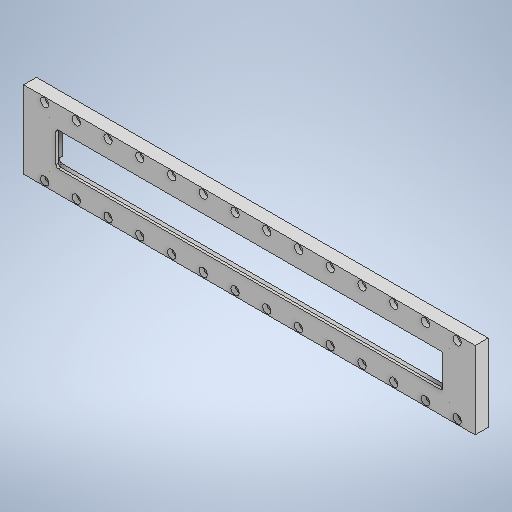
# Autodesk Inventor part: Bauteil4
Saved by Autodesk Inventor 2025.2 (Build 292293000, 293)
## iProperties
Created: 2025-01-07
Part Number: Bauteil4
Material: Generisch
Document SubType Name: Modeling
Designer: gorenfl4
Density: 1 g/cm^3
Appearance: Vorgabe
Author: gorenfl4
Autodesk Inventor part; units mm, degrees
ref_plane "YZ Plane" through (0, 0, 0) normal (1, 0, 0) x (0, 1, 0)
ref_plane "XZ Plane" through (0, 0, 0) normal (0, 1, 0) x (-1, 0, 0)
ref_plane "XY Plane" through (0, 0, 0) normal (0, 0, 1) x (1, 0, 0)
sketch "Skizze1" plane through (0, 0, 0) normal (0, 1, 0) x (-1, 0, 0)
  line L0 (0, 42.9058) -> (-350, 42.9058)
  line L1 (-350, 42.9058) -> (-350, -17.0942)
  line L2 (-350, -17.0942) -> (0, -17.0942)
  line L3 (0, -17.0942) -> (0, 42.9058)
  point P0 (0, 0)
  dimension "d0" = 350
  dimension "d1" = 0
  dimension "d2" = 60
  constraints: 8 end point, 2 parallel, 1 horizontal, 1 perpendicular
  measures "d0" distance from line of point (0, 0) L1
  measures "d1" distance from line of point (0, 0) L3
  measures "d2" distance between parallel lines of L0 L2
extrude "Extrusion1" add sketch "Skizze1" along normal blind 10
sketch "Skizze2" plane through (0, 10, 0) normal (0, 1, 0) x (1, 0, 0)
  line L0 (25, 0.0942) -> (325, 0.0942)
  line L1 (325, 0.0942) -> (325, -25.9058)
  line L2 (325, -25.9058) -> (25, -25.9058)
  line L3 (25, -25.9058) -> (25, 0.0942)
  line L4 (0, 17.0942) -> (0, -42.9058) projected
  line L5 (350, -42.9058) -> (350, 17.0942) projected
  line L6 (350, 17.0942) -> (0, 17.0942) projected
  line L7 (0, -42.9058) -> (350, -42.9058) projected
  point P0 (0, 0)
  point P1 (175, 17.0942)
  dimension "d5" = 25
  dimension "d6" = 25
  dimension "d7" = 17
  dimension "d8" = 17
  constraints: 8 end point, 2 parallel, 1 horizontal, 1 midpoint, 1 perpendicular
  measures "d5" distance between parallel lines of L4 L3
  measures "d6" distance between parallel lines of L5 L1
  measures "d7" distance from line of point (175, 17.094) L0
  measures "d8" distance between parallel lines of L7 L2
extrude "Extrusion2" cut sketch "Skizze2" against normal through all contours L0 L1 L2 L3
fillet "Rundung1" radius 2 1 edges at (25, 5, -0.0942)
fillet "Rundung2" radius 2 1 edges at (25, 5, 25.9058)
fillet "Rundung3" radius 2 1 edges at (325, 5, -0.0942)
fillet "Rundung4" radius 2 1 edges at (325, 5, 25.9058)
sketch "Skizze4" plane through (0, 10, 0) normal (0, 1, 0) x (1, 0, 0)
  line L0 (20, -30.9058) -> (330, -30.9058)
  line L1 (330, 5.0942) -> (20, 5.0942)
  line L2 (25, -23.9058) -> (25, -1.9058) projected
  line L3 (323, -25.9058) -> (27, -25.9058) projected
  line L4 (27, 0.0942) -> (323, 0.0942) projected
  line L5 (325, -1.9058) -> (325, -23.9058) projected
  arc A0 (20, 5.0942) -> (20, 0.0942) centre (20, 2.5942) ccw
  arc A1 (20, -25.9058) -> (20, -30.9058) centre (20, -28.4058) ccw
  arc A2 (330, 0.0942) -> (330, 5.0942) centre (330, 2.5942) ccw
  arc A3 (330, -30.9058) -> (330, -25.9058) centre (330, -28.4058) ccw
  line L6 (330, 0.0942) -> (330, -25.9058)
  line L7 (20, 0.0942) -> (20, -25.9058)
  point P0 (0, 0)
  dimension "d32" = 5
  dimension "d33" = 5
  dimension "d110" = 2.5
  dimension "d111" = 2.5
  dimension "d112" = 2.5
  dimension "d113" = 2.5
  dimension "d114" = 5
  dimension "d115" = 5
  constraints: 8 end point, 8 point on circle, 4 centre point, 4 line through centre, 4 tangent, 1 horizontal, 1 parallel, 1 vertical
  measures "d32" distance between parallel lines of L0 L3
  measures "d33" distance between parallel lines of L4 L1
  measures "d110" radius of A0
  measures "d111" radius of A1
  measures "d112" radius of A2
  measures "d113" radius of A3
  measures "d114" distance between parallel lines of L5 L6
  measures "d115" distance between parallel lines of L7 L2
extrude "Extrusion4" cut sketch "Skizze4" against normal blind 8
sketch "Skizze14" plane through (0, 0, 0) normal (0, -1, 0) x (1, 0, 0)
  line L0 (0, 42.9058) -> (350, 42.9058) projected
  line L1 (0, -17.0942) -> (0, 42.9058) projected
  point P0 (0, 0)
  point P1 (16.3, 39.1558)
  dimension "d116" = 3.75
  dimension "d117" = 16.3
  measures "d116" distance from line of L0 point (16.3, 39.156)
  measures "d117" distance from line of L1 point (16.3, 39.156)
hole "Bohrung8" at (16.3, 0, 39.1558) direction (0, 1, 0) diameter 3.4 end through all counterbore diameter 6.5 counterbore depth 3.4 clearance for "Inbusschraube DIN EN ISO 4762" size "M3" standard "DIN"
pattern_linear "Rechteckige Anordnung2" count 14 spacing 24.6 along (1, 0, 0) count 2 spacing 52.5 along (0, 0, -1) of "Bohrung8"
equation "\"d7\" = d8"
equation "\"d32\" = d33"
equation "\"d114\" = d33"
equation "\"d115\" = d33"
